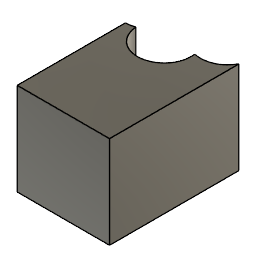
drawer container (Autodesk Fusion 360 design; units mm, degrees)
part number: 2026-07-15-00-17-15-300
part number: 2026-07-15-18-52-34-244
Autodesk Fusion 360 part; units mm, degrees
note: some values were not read from the file. Chosen so that the rebuilt part matches the saved one: which bodies a step acts on.
sketch "Sketch1" plane through (0, 0, 0) normal (0, 0, 1) x (1, 0, 0)
sketch "Sketch2" plane through (0, 0, 0) normal (1, 0, 0) x (0, 1, 0)
  line L0 (-150, -80) -> (-10.0019, -80)
  line L1 (-10.0019, -80) -> (-10.0019, 20)
  line L2 (-10.0019, 20) -> (-150, 20)
  line L3 (-150, 20) -> (-150, -80)
  dimension "d3" = 100
  constraint horizontal L0
  constraint vertical L1
  constraint horizontal L2
  constraint vertical L3
  measures "d3" distance of L0.start L2.end
extrude "Extrude1" add sketch "Sketch2" along normal blind 100 makes body 1
move_body "Move1" bodies 1 to x (1, 0, 0) y (0, 1, 0) z (0, 0, 1) at (-26.9375, -6.5143, 74.6237)
sketch "Sketch1 (2)" plane through (0, 0, 0) normal (0, 0, 1) x (1, 0, 0) in component "pen holder"
sketch "Sketch2 (2)" plane through (0, 0, 0) normal (0, 0, 1) x (1, 0, 0) in component "pen holder"
  spline S0 degree 4 poles (-37.1693, 44.8929, 2.0524) (-49.827, 67.9335, 2.0524) (-85.2233, 67.6007, 2.0524) (-100.346, 38.962, 2.0524) (-86.7187, 15.2963, 2.0524) knots 0.11903345 0.11903345 0.11903345 0.11903345 0.11903345 0.90124376 0.90124376 0.90124376 0.90124376 0.90124376
  line L0 (-37.1693, 44.8929, 2.0524) -> (-49.827, 67.9335, 2.0524) construction
  line L1 (-49.827, 67.9335, 2.0524) -> (-85.2233, 67.6007, 2.0524) construction
  line L2 (-85.2233, 67.6007, 2.0524) -> (-100.346, 38.962, 2.0524) construction
  line L3 (-100.346, 38.962, 2.0524) -> (-86.7187, 15.2963, 2.0524) construction
  spline S1 degree 4 poles (5.2991, 5.9786, 2.0524) (22.0769, 25.1322, 2.0524) (10.9529, 56.8319, 2.0524) (-18.9169, 62.817, 2.0524) (-37.1693, 44.8929, 2.0524) knots 0.11903345 0.11903345 0.11903345 0.11903345 0.11903345 0.87667324 0.87667324 0.87667324 0.87667324 0.87667324
  line L4 (5.2991, 5.9786, 2.0524) -> (22.0769, 25.1322, 2.0524) construction
  line L5 (22.0769, 25.1322, 2.0524) -> (10.9529, 56.8319, 2.0524) construction
  line L6 (10.9529, 56.8319, 2.0524) -> (-18.9169, 62.817, 2.0524) construction
  line L7 (-18.9169, 62.817, 2.0524) -> (-37.1693, 44.8929, 2.0524) construction
  spline S2 degree 4 poles (-16.7433, -47.2381, 2.0524) (6.9935, -56.4531, 2.0524) (32.9769, -35.158, 2.0524) (28.3849, -5.0425, 2.0524) (5.2991, 5.9786, 2.0524) knots 0.11903345 0.11903345 0.11903345 0.11903345 0.11903345 0.87667324 0.87667324 0.87667324 0.87667324 0.87667324
  line L8 (-16.7433, -47.2381, 2.0524) -> (6.9935, -56.4531, 2.0524) construction
  line L9 (6.9935, -56.4531, 2.0524) -> (32.9769, -35.158, 2.0524) construction
  line L10 (32.9769, -35.158, 2.0524) -> (28.3849, -5.0425, 2.0524) construction
  line L11 (28.3849, -5.0425, 2.0524) -> (5.2991, 5.9786, 2.0524) construction
  spline S3 degree 4 poles (-73.9661, -40.9267, 2.0524) (-78.0196, -68.1676, 2.0524) (-47.9272, -88.3743, 2.0524) (-19.2943, -73.6355, 2.0524) (-16.7433, -47.2381, 2.0524) knots 0.09122943 0.09122943 0.09122943 0.09122943 0.09122943 0.87667324 0.87667324 0.87667324 0.87667324 0.87667324
  line L12 (-73.9661, -40.9267, 2.0524) -> (-78.0196, -68.1676, 2.0524) construction
  line L13 (-78.0196, -68.1676, 2.0524) -> (-47.9272, -88.3743, 2.0524) construction
  line L14 (-47.9272, -88.3743, 2.0524) -> (-19.2943, -73.6355, 2.0524) construction
  line L15 (-19.2943, -73.6355, 2.0524) -> (-16.7433, -47.2381, 2.0524) construction
  spline S4 degree 4 poles (-86.7187, 15.2963, 2.0524) (-112.6303, 10.0184, 2.0524) (-122.4235, -23.7935, 2.0524) (-100.0123, -46.4016, 2.0524) (-73.9661, -40.9267, 2.0524) knots 0.11032757 0.11032757 0.11032757 0.11032757 0.11032757 0.88740085 0.88740085 0.88740085 0.88740085 0.88740085
  line L16 (-86.7187, 15.2963, 2.0524) -> (-112.6303, 10.0184, 2.0524) construction
  line L17 (-112.6303, 10.0184, 2.0524) -> (-122.4235, -23.7935, 2.0524) construction
  line L18 (-122.4235, -23.7935, 2.0524) -> (-100.0123, -46.4016, 2.0524) construction
  line L19 (-100.0123, -46.4016, 2.0524) -> (-73.9661, -40.9267, 2.0524) construction
  circle A0 through (-8.1136, -7.4617, -54.9375) (-60.6136, 22.8492, -54.9375) (-60.6136, -37.7726, -54.9375)
  dimension "d24" = 70
sketch "Sketch2 (2) (curves 2.0524 mm off its plane)" plane through (0, 0, 2.0524) normal (0, 0, 1) x (1, 0, 0)
  spline S0 degree 4 poles (-37.1693, 44.8929) (-49.827, 67.9335) (-85.2233, 67.6007) (-100.346, 38.962) (-86.7187, 15.2963) knots 0.119033 0.119033 0.119033 0.119033 0.119033 0.901244 0.901244 0.901244 0.901244 0.901244
  line L0 (-37.1693, 44.8929) -> (-49.827, 67.9335) construction
  line L1 (-49.827, 67.9335) -> (-85.2233, 67.6007) construction
  line L2 (-85.2233, 67.6007) -> (-100.346, 38.962) construction
  line L3 (-100.346, 38.962) -> (-86.7187, 15.2963) construction
  spline S1 degree 4 poles (5.2991, 5.9786) (22.0769, 25.1322) (10.9529, 56.8319) (-18.9169, 62.817) (-37.1693, 44.8929) knots 0.119033 0.119033 0.119033 0.119033 0.119033 0.876673 0.876673 0.876673 0.876673 0.876673
  line L4 (5.2991, 5.9786) -> (22.0769, 25.1322) construction
  line L5 (22.0769, 25.1322) -> (10.9529, 56.8319) construction
  line L6 (10.9529, 56.8319) -> (-18.9169, 62.817) construction
  line L7 (-18.9169, 62.817) -> (-37.1693, 44.8929) construction
  spline S2 degree 4 poles (-16.7433, -47.2381) (6.9935, -56.4531) (32.9769, -35.158) (28.3849, -5.0425) (5.2991, 5.9786) knots 0.119033 0.119033 0.119033 0.119033 0.119033 0.876673 0.876673 0.876673 0.876673 0.876673
  line L8 (-16.7433, -47.2381) -> (6.9935, -56.4531) construction
  line L9 (6.9935, -56.4531) -> (32.9769, -35.158) construction
  line L10 (32.9769, -35.158) -> (28.3849, -5.0425) construction
  line L11 (28.3849, -5.0425) -> (5.2991, 5.9786) construction
  spline S3 degree 4 poles (-73.9661, -40.9267) (-78.0196, -68.1676) (-47.9272, -88.3743) (-19.2943, -73.6355) (-16.7433, -47.2381) knots 0.091229 0.091229 0.091229 0.091229 0.091229 0.876673 0.876673 0.876673 0.876673 0.876673
  line L12 (-73.9661, -40.9267) -> (-78.0196, -68.1676) construction
  line L13 (-78.0196, -68.1676) -> (-47.9272, -88.3743) construction
  line L14 (-47.9272, -88.3743) -> (-19.2943, -73.6355) construction
  line L15 (-19.2943, -73.6355) -> (-16.7433, -47.2381) construction
  spline S4 degree 4 poles (-86.7187, 15.2963) (-112.6303, 10.0184) (-122.4235, -23.7935) (-100.0123, -46.4016) (-73.9661, -40.9267) knots 0.110328 0.110328 0.110328 0.110328 0.110328 0.887401 0.887401 0.887401 0.887401 0.887401
  line L16 (-86.7187, 15.2963) -> (-112.6303, 10.0184) construction
  line L17 (-112.6303, 10.0184) -> (-122.4235, -23.7935) construction
  line L18 (-122.4235, -23.7935) -> (-100.0123, -46.4016) construction
  line L19 (-100.0123, -46.4016) -> (-73.9661, -40.9267) construction
extrude "Extrude11" add sketch "Sketch2 (2) (curves 2.0524 mm off its plane)" along normal blind 150 separate body makes body 2 in component "pen holder"
sketch "Sketch2 (2) (curves -54.9375 mm off its plane)" plane through (0, 0, -54.9375) normal (0, 0, 1) x (1, 0, 0)
  circle A0 centre (-43.1136, -7.4617) radius 35
extrude "Extrude12" cut sketch "Sketch2 (2) (curves -54.9375 mm off its plane)" along normal blind 200 bodies 2 in component "pen holder"
move_body "Move1'" bodies 2 to x (-1, 0, 0) y (0, 1, 0) z (0, 0, -1) at (-33.4866, 0, 304.1047) in component "pen holder"
move_body "Move2" bodies 2 to x (1, 0, 0) y (0, 1, 0) z (0, 0, 1) at (0, 0, -160) in component "pen holder"
move_body "Move2'" bodies 1 to x (1, 0, 0) y (0, 1, 0) z (0, 0, 1) at (-0.6573, -0.0909, 1.1243)
move_body "Move3" bodies 1 to x (1, 0, 0) y (0, 1, 0) z (0, 0, 1) at (1.5449, 5.4785, -0.0439)
combine "Combine1" operation cut target body 1 tool bodies 2 body 2 seen with x (1, 0, 0) y (0, 1, 0) z (0, 0, 1) at (0.2658, 15.1802, 3.9714) makes body 3 at (7.2835, -104.4607, -4.2959)
delete_body "RemoveBody1" bodies 1
sketch "Sketch3" plane through (-26.0498, 0, 0) normal (-1, 0, 0) x (0, -1, 0)
  line L0 (34.0027, -3.9762) -> (11.1286, -3.9762)
  line L1 (11.1286, -3.9762) -> (11.1286, -4.2959)
  line L2 (11.1286, -4.2959) -> (151.1267, -4.2959)
  line L3 (151.1267, -4.2959) -> (151.1267, 95.7041)
  line L4 (151.1267, 95.7041) -> (34.0027, 95.7041)
  line L5 (34.0027, 95.7041) -> (34.0027, -3.9762)
  line L6 (60, 70) -> (140, 70)
  line L7 (140, 70) -> (140, 10)
  line L8 (140, 10) -> (60, 10)
  line L9 (60, 10) -> (60, 70)
  constraint horizontal L6
  constraint vertical L7
  constraint horizontal L8
  constraint vertical L9
extrude "Extrude2" cut sketch "Sketch3" against normal blind 90 contours L6 L7 L8 L9 bodies 3
component "pen holder" placed x (1, 0, 0) y (0, 1, 0) z (0, 0, 1) at (0.2658, 15.1802, 3.9714)
